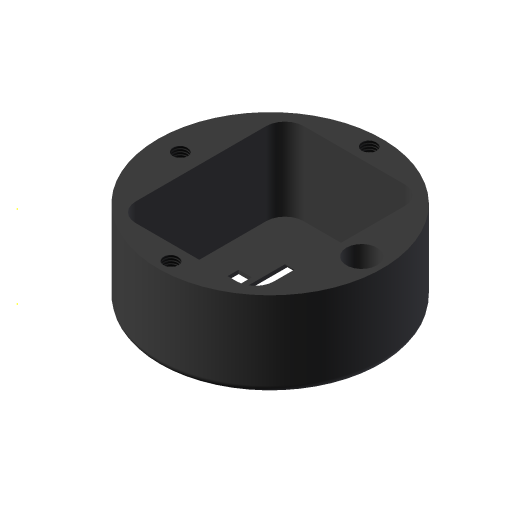
# Autodesk Inventor part: webcam_holder_center
Saved by Autodesk Inventor 2023 (Build 270158000, 158)
## iProperties
Created: 2024-01-25
Part Number: webcam_holder_center
Material: Generic
Document SubType Name: Modeling
Designer: qg3473
Density: 1 g/cm^3
Appearance: Default
Author: qg3473
Autodesk Inventor part; units mm, degrees
ref_plane "YZ Plane" through (0, 0, 0) normal (1, 0, 0) x (0, 1, 0)
ref_plane "XZ Plane" through (0, 0, 0) normal (0, 1, 0) x (-1, 0, 0)
ref_plane "XY Plane" through (0, 0, 0) normal (0, 0, 1) x (1, 0, 0)
sketch "Sketch1" plane through (0, 0, 0) normal (0, 1, 0) x (-1, 0, 0)
  point P0 (0, 0)
sketch "Sketch2" plane through (0, 0, 0) normal (0, 1, 0) x (-1, 0, 0)
  line L0 (-14.0823, -12.5349) -> (-51.0823, -12.5349)
  line L1 (-51.0823, -12.5349) -> (-51.0823, -57.4349)
  line L2 (-51.0823, -57.4349) -> (-14.0823, -57.4349)
  line L3 (-14.0823, -57.4349) -> (-14.0823, -12.5349)
  circle A0 centre (-32.5823, -34.9849) radius 30
  point P0 (0, 0)
  dimension "d0" = 37
  dimension "d1" = 44.9
  constraints: 8 end point, 2 parallel, 1 centre point, 1 horizontal, 1 perpendicular
  measures "d0" distance of L2.end L1.end
  measures "d1" distance of L1.end L0.end
extrude "Extrusion1" add sketch "Sketch2" against normal blind 1 contours L3 L2 L1 L0 | A0
extrude "Extrusion2" add sketch "Sketch2" along normal blind 22
sketch "Sketch3" plane through (32.5823, 22, -34.9849) normal (0, 1, 0) x (1, 0, 0)
  circle A0 centre (24.4505, 0.0199) radius 4.09
  point P0 (-32.5823, -34.9849)
  dimension "d9" = 8.18
  constraints: 1 centre point
  measures "d9" diameter of A0
extrude "Extrusion3" cut sketch "Sketch3" against normal up to next
sketch "Sketch4" plane through (32.5823, 22, -34.9849) normal (0, 1, 0) x (1, 0, 0)
  point P0 (-32.5823, -34.9849)
sketch "Sketch6" plane through (32.5823, 22, -34.9849) normal (0, 1, 0) x (1, 0, 0)
  circle A0 centre (0, 0) radius 30 projected
  line L0 (-30, 0) -> (-24, 0)
  circle A1 centre (-24, 0) radius 2
  point P0 (-32.5823, -34.9849)
  dimension "d23" = 6
  dimension "d24" = 4
  constraints: 2 end point, 1 centre point, 1 coincident, 1 horizontal, 1 horizontal alignment, 1 other
  measures "d23" distance of L0.start L0.end
  measures "d24" diameter of A1
sketch "Sketch7" plane through (32.5823, 22, -34.9849) normal (0, 1, 0) x (1, 0, 0)
  circle A0 centre (0, 0) radius 30 projected
  line L0 (0, -30) -> (0, -26.5)
  circle A1 centre (0, -26.5) radius 2
  line L1 (0, 30) -> (0, 26.5)
  circle A2 centre (0, 26.5) radius 2
  point P0 (-32.5823, -34.9849)
  dimension "d25" = 3.5
  dimension "d26" = 4
  dimension "d27" = 3.5
  dimension "d28" = 4
  constraints: 4 end point, 2 centre point, 2 coincident, 2 point on circle, 2 vertical
  measures "d25" distance of L0.start L0.end
  measures "d26" diameter of A1
  measures "d27" distance of L1.start L1.end
  measures "d28" diameter of A2
extrude "Extrusion5" cut sketch "Sketch7" against normal blind 10 contours A2 | A1
extrude "Extrusion6" cut sketch "Sketch6" against normal blind 10 contours A1
thread "Thread4" size "M4x0.7" class "6H" standard "ANSI Metric M Profile" length 10
thread "Thread5" size "M4x0.7" class "6H" standard "ANSI Metric M Profile" full length
thread "Thread6" size "M4x0.7" class "6H" standard "ANSI Metric M Profile" full length
sketch "Sketch8" plane through (32.5823, 22, -34.9849) normal (0, 1, 0) x (1, 0, 0)
  point P0 (-32.5823, -34.9849)
fillet "Fillet1" radius 2 1 edges at (62.5823, -1, -34.9849)
fillet "Fillet2" radius 5 4 edges at (14.0823, 11, -57.4349) (14.0823, 11, -12.5349) (51.0823, 11, -12.5349) (51.0823, 11, -57.4349)
sketch "Sketch10" plane through (0, -1, 0) normal (0, -1, 0) x (1, 0, 0)
  line L0 (38.5823, -44.9849) -> (26.5823, -44.9849)
  line L1 (26.5823, -44.9849) -> (26.5823, -24.9849)
  line L2 (26.5823, -24.9849) -> (38.5823, -24.9849)
  line L3 (38.5823, -24.9849) -> (38.5823, -44.9849)
  arc A0 (60.4997, -32.8347) -> (60.4961, -37.1806) centre (32.5823, -34.9849) ccw projected
  line L4 (38.5823, -44.9849) -> (26.5823, -24.9849) construction
  line L5 (26.5823, -44.9849) -> (38.5823, -24.9849) construction
  line L6 (43.6176, -37.4849) -> (40.1176, -37.4849)
  line L7 (40.1176, -37.4849) -> (40.1176, -32.4849)
  line L8 (40.1176, -32.4849) -> (43.6176, -32.4849)
  line L9 (43.6176, -32.4849) -> (43.6176, -37.4849)
  line L10 (43.6176, -37.4849) -> (40.1176, -32.4849) construction
  line L11 (40.1176, -37.4849) -> (43.6176, -32.4849) construction
  line L12 (25.1564, -37.4849) -> (21.6564, -37.4849)
  line L13 (21.6564, -37.4849) -> (21.6564, -32.4849)
  line L14 (21.6564, -32.4849) -> (25.1564, -32.4849)
  line L15 (25.1564, -32.4849) -> (25.1564, -37.4849)
  line L16 (25.1564, -37.4849) -> (21.6564, -32.4849) construction
  line L17 (21.6564, -37.4849) -> (25.1564, -32.4849) construction
  point P0 (0, 0)
  point P1 (41.8676, -34.9849)
  point P2 (23.4064, -34.9849)
  dimension "d49" = 12
  dimension "d50" = 20
  dimension "d51" = 3.5
  dimension "d52" = 5
  dimension "d53" = 3.5
  dimension "d54" = 5
  constraints: 36 end point, 6 midpoint, 6 parallel, 3 horizontal, 3 perpendicular
  measures "d49" distance of L1.end L2.end
  measures "d50" distance of L0.end L1.end
  measures "d51" distance of L7.end L8.end
  measures "d52" distance of L6.end L7.end
  measures "d53" distance of L13.end L14.end
  measures "d54" distance of L12.end L13.end
extrude "Extrusion8" cut sketch "Sketch10" against normal blind 2
fillet "Fillet3" radius 1 2 edges at (32.5823, -1, -44.9849) (32.5823, -1, -24.9849)
body "Solid1"
